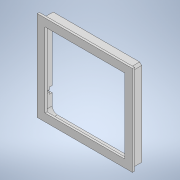
# Autodesk Inventor part: Sand Cover
Saved by Autodesk Inventor 2022 (Build 260153000, 153)
## iProperties
Created: 2022-05-29
Part Number: Sand Cover
Material: Generic
Document SubType Name: Modeling
Designer: Nick
Density: 1 g/cm^3
Appearance: Default
Author: Nick
Autodesk Inventor part; units mm, degrees
ref_plane "YZ Plane" through (0, 0, 0) normal (1, 0, 0) x (0, 1, 0)
ref_plane "XZ Plane" through (0, 0, 0) normal (0, 1, 0) x (-1, 0, 0)
ref_plane "XY Plane" through (0, 0, 0) normal (0, 0, 1) x (1, 0, 0)
sketch "Sketch1" plane through (0, 0, 0) normal (0, 0, 1) x (1, 0, 0)
  line L0 (0, 0) -> (185, 0)
  line L1 (185, 0) -> (185, 175)
  line L2 (185, 175) -> (0, 175)
  line L3 (0, 175) -> (0, 0)
  line L4 (15, 160) -> (170, 160)
  line L5 (170, 160) -> (170, 15)
  line L6 (170, 15) -> (15, 15)
  line L7 (15, 15) -> (15, 160)
  dimension "d0" = 185
  dimension "d1" = 175
  dimension "d2" = 15
  constraints: 16 end point, 4 parallel, 2 perpendicular, 1 horizontal, 3 other
  measures "d0" distance of L2.end L1.end
  measures "d1" distance of L1.end L0.end
  measures "d2" distance between parallel lines of L2 L4
extrude "Extrusion1" add sketch "Sketch1" along normal blind 4
sketch "Sketch2" plane through (0, 0, 0) normal (0, 0, -1) x (-1, 0, 0)
  line L0 (-185, 0) -> (-185, 175) projected
  line L1 (0, 0) -> (-185, 0) projected
  line L2 (0, 175) -> (0, 0) projected
  line L3 (-185, 175) -> (0, 175) projected
  line L4 (-15, 160) -> (-170, 160) projected
  line L5 (-15, 15) -> (-15, 160) projected
  line L6 (-170, 15) -> (-15, 15) projected
  line L7 (-170, 160) -> (-170, 15) projected
  line L8 (-2, 2) -> (-183, 2)
  line L9 (-183, 2) -> (-183, 173)
  line L10 (-183, 173) -> (-2, 173)
  line L11 (-2, 173) -> (-2, 2)
  line L12 (-4, 4) -> (-181, 4)
  line L13 (-181, 4) -> (-181, 171)
  line L14 (-181, 171) -> (-4, 171)
  line L15 (-4, 171) -> (-4, 4)
  line L16 (-9, 4) -> (-9, 171)
  line L17 (0, 0) -> (-7, 0)
  line L18 (-7, 0) -> (-7, 30)
  line L19 (-7, 30) -> (0, 30)
  line L20 (0, 30) -> (0, 0)
  line L21 (0, 175) -> (0, 0) projected
  line L22 (0, 175) -> (-7, 175)
  line L23 (-7, 175) -> (-7, 145)
  line L24 (-7, 145) -> (0, 145)
  line L25 (0, 145) -> (0, 175)
  line L26 (0, 54.5) -> (-7, 54.5)
  line L27 (-7, 54.5) -> (-7, 62.5)
  line L28 (-7, 62.5) -> (0, 62.5)
  line L29 (0, 62.5) -> (0, 54.5)
  line L30 (0, 112.5) -> (-7, 112.5)
  line L31 (-7, 112.5) -> (-7, 120.5)
  line L32 (-7, 120.5) -> (0, 120.5)
  line L33 (0, 120.5) -> (0, 112.5)
  line L34 (0, 175) -> (0, 0) projected
  point P0 (-7, 173)
  point P1 (-7, 2)
  point P2 (-2, 30)
  point P3 (-2, 145)
  point P4 (-7, 58.5)
  point P5 (-7, 116.5)
  point P6 (-2, 54.5)
  point P7 (-2, 62.5)
  point P8 (-2, 112.5)
  point P9 (-2, 120.5)
  dimension "d5" = 2
  dimension "d6" = 2
  dimension "d13" = 5
  dimension "d15" = 2
  dimension "d16" = 2
  dimension "d17" = 30
  dimension "d18" = 30
  dimension "d19" = 56.5
  dimension "d20" = 56.5
  dimension "d21" = 8
  dimension "d22" = 8
  constraints: 50 end point, 8 parallel, 4 collinear, 4 horizontal, 4 perpendicular, 2 midpoint, 2 point on line, 1 vertical, 6 other
  measures "d5" distance between parallel lines of L2 L11
  measures "d6" distance between parallel lines of L11 L15
  measures "d13" distance between parallel lines of L15 L16
  measures "d15" distance between parallel lines of L16 L18
  measures "d16" distance between parallel lines of L16 L23
  measures "d17" distance of L17.end L18.end
  measures "d18" distance of L22.end L23.end
  measures "d19" distance from line of L8 point (-7, 58.5)
  measures "d20" distance from line of L10 point (-7, 116.5)
  measures "d21" distance of L26.end L27.end
  measures "d22" distance of L30.end L31.end
extrude "Extrusion2" add sketch "Sketch2" along normal blind 16 contours L8 L9 L10 L23 L14 L13 L12 L18 | L12 L16 L14 L23 L24 L15 L32 L31 L30 L28 L27 L26 L19 L18 | L19 L15 L26 L11 | L11 L32 L15 L24 | L28 L15 L30 L11
fillet "Fillet1" radius 20 2 edges at (181, 4, -8) (181, 171, -8)
fillet "Fillet2" radius 10 2 edges at (9, 4, -8) (9, 171, -8)
chamfer "Chamfer1" distance 4 angle 45 4 edges at (183, 2, -8) (183, 173, -8) (7, 2, -8) (7, 173, -8)
sketch "Sketch3" plane through (0, 0, -16) normal (0, 0, -1) x (-1, 0, 0)
  line L0 (-2, 54.5) -> (-2, 30) projected
  line L1 (-9, 14) -> (-9, 161) projected
  line L2 (-2, 36.25) -> (-9, 36.25)
  line L3 (-9, 36.25) -> (-9, 48.25)
  line L4 (-9, 48.25) -> (-2, 48.25)
  line L5 (-2, 48.25) -> (-2, 36.25)
  point P0 (0, 0)
  point P1 (-2, 42.25)
  point P2 (-2, 48.25)
  dimension "d24" = 12
  constraints: 8 end point, 2 midpoint, 2 parallel, 2 point on line, 1 horizontal, 1 perpendicular
  measures "d24" distance of L2.end L3.end
extrude "Extrusion3" cut sketch "Sketch3" against normal blind 5
sketch "Sketch4" plane through (9, 14, 0) normal (1, 0, 0) x (0, 0, -1)
  line L0 (11, 34.25) -> (16, 34.25) projected
  line L1 (16, 147) -> (16, 34.25) projected
  line L2 (0, 147) -> (16, 147) projected
  line L3 (0, 0) -> (0, 147) projected
  line L4 (16, 0) -> (0, 0) projected
  line L5 (16, 22.25) -> (16, 0) projected
  line L6 (16, 22.25) -> (11, 22.25) projected
  line L7 (11, 22.25) -> (11, 34.25) projected
  line L8 (11, 22.25) -> (11, 34.25) projected
  line L9 (11, 26.25) -> (0, 26.25)
  line L10 (0, 26.25) -> (0, 30.25)
  line L11 (0, 30.25) -> (11, 30.25)
  line L12 (11, 30.25) -> (11, 26.25)
  point P0 (0, -14)
  point P1 (11, 28.25)
  point P2 (0, 30.25)
  point P3 (0, 26.25)
  dimension "d27" = 4
  constraints: 8 end point, 2 midpoint, 2 parallel, 1 collinear, 1 horizontal, 1 perpendicular, 1 point on line
  measures "d27" distance between parallel lines of L11 L9
extrude "Extrusion4" cut sketch "Sketch4" against normal blind 3 contours L7 L9 L3 L11
equation "\"d18\" = d17"
equation "\"d20\" = d19"
equation "\"d22\" = d21"
body "Solid1"
